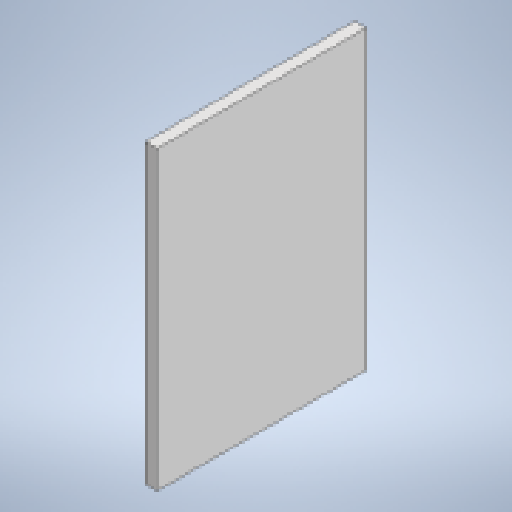
# Autodesk Inventor part: Y_PLATE
Saved by Autodesk Inventor 2023 (Build 270158000, 158)
## iProperties
Created: 2022-05-03
Part Number: Y_PLATE
Material: Generic
Document SubType Name: Modeling
Designer: plebbb
Density: 1 g/cm^3
Appearance: Default
Author: plebbb
Autodesk Inventor part; units mm, degrees
ref_plane "YZ Plane" through (0, 0, 0) normal (1, 0, 0) x (0, 1, 0)
ref_plane "XZ Plane" through (0, 0, 0) normal (0, 1, 0) x (-1, 0, 0)
ref_plane "XY Plane" through (0, 0, 0) normal (0, 0, 1) x (1, 0, 0)
sketch "Sketch1" plane through (0, 0, 0) normal (1, 0, 0) x (0, 1, 0)
  line L0 (0, 0) -> (215.9, 0)
  line L1 (215.9, 0) -> (215.9, -152.4)
  line L2 (215.9, -152.4) -> (0, -152.4)
  line L3 (0, -152.4) -> (0, 0)
  dimension "d0" = 152.4
  dimension "d1" = 215.9
  constraints: 8 end point, 2 parallel, 1 horizontal, 1 perpendicular
  measures "d0" distance of L2.end L0.start
  measures "d1" distance of L1.end L2.end
extrude "Extrusion1" add sketch "Sketch1" along normal blind 8.4667
sketch "Sketch3" plane through (8.4667, 0, 0) normal (1, 0, 0) x (0, 0, -1)
  line L0 (121.2, 175.9) -> (31.2, 175.9) construction
  line L1 (31.2, 175.9) -> (31.2, 200.9) construction
  line L2 (31.2, 200.9) -> (121.2, 200.9) construction
  line L3 (121.2, 200.9) -> (121.2, 175.9) construction
  circle A0 centre (121.2, 175.9) radius 4
  circle A1 centre (31.2, 175.9) radius 4
  circle A2 centre (121.2, 200.9) radius 4
  circle A3 centre (31.2, 200.9) radius 4
  line L4 (152.4, 215.9) -> (0, 215.9) construction
  point P0 (0, 0)
  point P1 (76.2, 175.9)
  point P2 (76.2, 215.9)
  point P3 (76.2, 215.9)
  dimension "d4" = 8
  dimension "d5" = 25
  dimension "d6" = 90
  dimension "d7" = 15
  constraints: 8 end point, 4 centre point, 4 coincident, 3 equal radius, 3 midpoint, 2 parallel, 1 horizontal, 1 perpendicular, 1 vertical alignment
  measures "d4" diameter of A0
  measures "d5" distance of L0.end L1.end
  measures "d6" distance of L0.start L0.end
  measures "d7" distance from line of point (76.2, 215.9) L2
extrude "Extrusion2" cut sketch "Sketch3" against normal blind 8.4667
body "Solid1"
